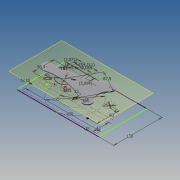
# Autodesk Inventor part: case A
Saved by Autodesk Inventor 2017 (Build 210142000, 142)
## iProperties
Part Number: case A
Material: Genérico
Document SubType Name: Modeling
Designer: Leo
Density: 1 g/cm^3
Appearance: Valor por defecto
Author: Leo
Autodesk Inventor part; units mm, degrees
ref_plane "YZ Plane" through (0, 0, 0) normal (1, 0, 0) x (0, 1, 0)
ref_plane "XZ Plane" through (0, 0, 0) normal (0, 1, 0) x (-1, 0, 0)
sketch "Boceto1" plane through (0, 0, 0) normal (0, 0, 1) x (1, 0, 0)
  circle A0 centre (0, 0) radius 3.175
  circle A1 centre (0, 0) radius 10 construction
  circle A2 centre (59.2187, -32.3945) radius 57.5 construction
  line L0 (28.2, 28.2) -> (-28.2, 28.2) construction
  line L1 (-28.2, 28.2) -> (-28.2, -28.2) construction
  line L2 (-28.2, -28.2) -> (28.2, -28.2) construction
  line L3 (28.2, -28.2) -> (28.2, 28.2) construction
  line L4 (-2.7639, 9.6105) -> (43.3262, 22.8657) construction
  line L5 (4.1137, -48.8168) -> (-9.5835, -2.8561) construction
  circle A3 centre (0, 0) radius 20
  line L6 (-29.9105, -43.3945) -> (170.0895, -43.3945) construction
  line L7 (170.0895, -43.3945) -> (170.0895, -85.3945) construction
  line L8 (170.0895, -85.3945) -> (-29.9105, -85.3945) construction
  line L9 (-29.9105, -85.3945) -> (-29.9105, -43.3945) construction
  circle A4 centre (59.2187, -32.3945) radius 4
  line L10 (-21.8022, 18.2667) -> (-28.8733, 25.3378)
  arc A5 (-25.3378, 28.8733) -> (-28.8733, 25.3378) centre (-27.1055, 27.1055) ccw
  line L11 (-25.3378, 28.8733) -> (-18.2667, 21.8022)
  arc A6 (-21.8022, 18.2667) -> (-18.2667, 21.8022) centre (-20.0345, 20.0345) ccw
  line L12 (21.8022, -18.2667) -> (28.8733, -25.3378)
  arc A7 (25.3378, -28.8733) -> (28.8733, -25.3378) centre (27.1055, -27.1055) ccw
  line L13 (25.3378, -28.8733) -> (18.2667, -21.8022)
  arc A8 (21.8022, -18.2667) -> (18.2667, -21.8022) centre (20.0345, -20.0345) ccw
  line L14 (-18.2667, -21.8022) -> (-25.3378, -28.8733)
  arc A9 (-28.8733, -25.3378) -> (-25.3378, -28.8733) centre (-27.1055, -27.1055) ccw
  line L15 (-28.8733, -25.3378) -> (-21.8022, -18.2667)
  arc A10 (-18.2667, -21.8022) -> (-21.8022, -18.2667) centre (-20.0345, -20.0345) ccw
  line L16 (18.2667, 21.8022) -> (25.3378, 28.8733)
  arc A11 (28.8733, 25.3378) -> (25.3378, 28.8733) centre (27.1055, 27.1055) ccw
  line L17 (28.8733, 25.3378) -> (21.8022, 18.2667)
  arc A12 (18.2667, 21.8022) -> (21.8022, 18.2667) centre (20.0345, 20.0345) ccw
  line L18 (-20.0345, 20.0345) -> (-27.1055, 27.1055) construction
  line L19 (20.0345, 20.0345) -> (27.1055, 27.1055) construction
  line L20 (-43.0653, -32.3945) -> (161.5026, -32.3945) construction
  circle A13 centre (122.4642, -2.3945) radius 2
  circle A14 centre (122.4642, -62.3945) radius 2
  circle A15 centre (122.4642, -2.3945) radius 12.5 construction
  circle A16 centre (59.2187, -32.3945) radius 30 construction
  line L21 (119.864, -14.621) -> (65.4592, -3.0507) construction
  line L22 (-39.9105, 39.6055) -> (180.0895, 39.6055)
  line L23 (180.0895, 39.6055) -> (180.0895, -90.3945)
  line L24 (180.0895, -90.3945) -> (-39.9105, -90.3945)
  line L25 (-39.9105, -90.3945) -> (-39.9105, 39.6055)
  circle A17 centre (-10.5521, -38.0553) radius 2
  circle A18 centre (-10.5521, -38.0553) radius 12.5 construction
  circle A19 centre (59.2187, -32.3945) radius 11 construction
  point P0 (-28.2, 0)
  point P1 (0, -28.2)
  point P2 (70.0895, -90.3945)
  point P3 (70.0895, -85.3945)
  dimension "d15" = 25
  dimension "d17" = 60
  dimension "d0" = 6.35
  dimension "d1" = 56.4
  dimension "d2" = 67.5
  dimension "d3" = 40
  dimension "d4" = 200
  dimension "d5" = 42
  dimension "d6" = 8
  dimension "d7" = 3.0945
  dimension "d8" = 5
  dimension "d9" = 40.0689
  dimension "d10" = 10
  dimension "d11" = 54.2111
  dimension "d12" = 7.0711
  dimension "d13" = 4
  dimension "d14" = 115
  dimension "d16" = 60
  dimension "d18" = 5
  dimension "d19" = 10
  dimension "d20" = 22
  dimension "d21" = 130
  dimension "d22" = 10
  constraints: 52 end point, 23 tangent, 20 point on circle, 18 centre point, 11 parallel, 9 coincident, 8 perpendicular, 5 midpoint, 4 horizontal, 4 point on line, 4 vertical alignment, 3 collinear, 3 horizontal alignment, 2 equal radius, 11 other
  measures "d0" diameter of A0
  measures "d1" distance of L0.end L1.end
  measures "d2" distance of A2.centre point (0, 0)
  measures "d3" diameter of A3
  measures "d4" distance of L7.end L8.end
  measures "d5" distance of L6.end L7.end
  measures "d6" diameter of A4
  measures "d7" distance edge to line of A2 L0
  measures "d8" distance between parallel lines of L11 L10
  measures "d9" distance of L19.start L18.start
  measures "d10" distance of L18.start L18.end
  measures "d11" distance of L19.end L18.end
  measures "d12" horizontal distance of L18.start L18.end
  measures "d13" diameter of A13
  measures "d14" diameter of A2
  measures "d16" distance of point (122.464, -2.394) A14.centre
  measures "d18" distance between parallel lines of L24 L8
  measures "d19" distance edge to line of A5 L22
  measures "d20" diameter of A19
  measures "d21" distance of L22.end L23.end
  measures "d22" distance between parallel lines of L25 L9
ref_plane "Plano de trabajo1" through (0, 0, 38) normal (0, 0, 1) x (1, 0, 0)
sketch "Boceto2" plane through (0, 0, 38) normal (0, 0, 1) x (1, 0, 0)
  circle A0 centre (-10.5521, -38.0553) radius 2 projected
  circle A1 centre (122.4642, -2.3945) radius 2 projected
  circle A2 centre (122.4642, -62.3945) radius 2 projected
  circle A3 centre (59.2187, -32.3945) radius 4 projected
  arc A4 (130.9422, -11.8313) -> (116.2276, 8.6524) centre (122.4642, -2.3945) ccw
  arc A5 (115.237, -72.8203) -> (130.9422, -52.9577) centre (122.4642, -62.3945) ccw
  arc A6 (130.9422, -11.8313) -> (130.9422, -52.9577) centre (149.4162, -32.3945) ccw
  arc A7 (-10.6779, -25.3701) -> (-7.485, -50.3648) centre (-10.5521, -38.0553) ccw
  arc A8 (-10.6779, -25.3701) -> (116.2276, 8.6524) centre (-13.2901, 238.066) ccw
  arc A9 (115.237, -72.8203) -> (-7.485, -50.3648) centre (29.0791, -197.1105) ccw
  point P0 (0, 0)
  constraints: 12 point on circle, 6 centre point, 6 tangent, 3 concentric, 2 equal radius
extrude "Extrusión1" add sketch "Boceto2" along normal blind 4
